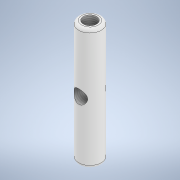
# Autodesk Inventor part: shaftorj
Saved by Autodesk Inventor 2020 (Build 240168000, 168)
## iProperties
Created: 2021-12-07
Part Number: shaftorj
Material: ABS Plastic
Document SubType Name: Modeling
Designer: Umur Batuhan Özmen
Density: 1.06 g/cm^3
Appearance: Smooth - White
Mass: 10.1137 g
Surface Area: 59.4598 cm^2
Volume: 9.54121 cm^3
Author: Umur Batuhan Özmen
## iProperties of the stored document _3DPrint.ipt
Created: 2021-12-10
Part Number: _3DPrint
Material: Generic
Document SubType Name: Modeling
Designer: Umur Batuhan Özmen
Density: 1 g/cm^3
Appearance: Default
Author: Umur Batuhan Özmen
Autodesk Inventor part; units mm, degrees
ref_plane "YZ Plane" through (0, 0, 0) normal (1, 0, 0) x (0, 1, 0)
ref_plane "XZ Plane" through (0, 0, 0) normal (0, 1, 0) x (-1, 0, 0)
sketch "Sketch1" plane through (0, 0, 0) normal (0, 1, 0) x (-1, 0, 0)
  circle A0 centre (0, 0) radius 7.5004
  constraints: 1 centre point, 1 coincident
extrude "Extrusion1" add sketch "Sketch1" along normal blind 80
sketch "Sketch2" plane through (0, 80, 0) normal (0, 1, 0) x (1, 0, 0)
  point P0 (0, 0)
hole "Hole1" at (0, 80, 0) direction (0, -1, 0) diameter 8.8 depth 30
thread "Thread1" size "M9x1.25" class "6H" standard "ISO Metric profile" length 30
hole "Hole2" at (0, 0, 0) direction (0, 1, 0) diameter 8.8 depth 30
sketch "Sketch6" plane through (0, 0, 0) normal (1, 0, 0) x (0, 1, 0)
  line L0 (0, -7.5004) -> (0, 7.5004) projected
  line L1 (0, -7.5004) -> (40, -7.5004)
  line L2 (0, -7.5004) -> (80, -7.5004) projected
  point P0 (0, 0)
  constraints: 2 end point, 1 midpoint
ref_plane "Work Plane1" through (0, 0, -7.5004) normal (0, 0, -1) x (-1, 0, 0)
sketch "Sketch7" plane through (0, 0, -7.5004) normal (0, 0, -1) x (-1, 0, 0)
  line L0 (0, 0) -> (0, 40)
  circle A0 centre (0, 40) radius 4.4
  dimension "d22" = 40
  dimension "d23" = 8.8
  constraints: 2 end point, 1 centre point, 1 coincident, 1 vertical
  measures "d22" distance of L0.start L0.end
  measures "d23" diameter of A0
hole "Hole3" at (0, 40, -7.5004) direction (0, 0, 1) diameter 9 end through all
thread "Thread3" size "M9x1.25" class "6H" standard "ANSI Metric M Profile" length 30
thread "Thread4" size "M9x1.25" class "6H" standard "ANSI Metric M Profile" length 30
fillet "Fillet1" radius 2 2 edges at (7.5004, 0, 0) (7.5004, 80, 0)
body "Solid1"
